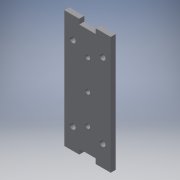
# Autodesk Inventor part: Tilt back support with counter balance option
Saved by Autodesk Inventor 2018 (Build 220112000, 112)
## iProperties
Created: 2018-06-26
Part Number: Tilt back support with counter balance option
Material: Generic
Document SubType Name: Modeling
Designer: Ajith Thomas
Density: 1 g/cm^3
Appearance: Default
Author: Ajith Thomas
Autodesk Inventor part; units mm, degrees
ref_plane "YZ Plane" through (0, 0, 0) normal (1, 0, 0) x (0, 1, 0)
ref_plane "XZ Plane" through (0, 0, 0) normal (0, 1, 0) x (-1, 0, 0)
ref_plane "XY Plane" through (0, 0, 0) normal (0, 0, 1) x (1, 0, 0)
sketch "Sketch1" plane through (0, 0, 0) normal (0, 0, 1) x (1, 0, 0)
  line L0 (5, 1.5) -> (-5, 1.5) projected
  line L1 (-5, 1.5) -> (-5, -1.5) projected
  line L2 (-5, -1.5) -> (5, -1.5) projected
  line L3 (5, -1.5) -> (5, 1.5) projected
  line L4 (5, -66.5) -> (-5, -66.5) projected
  line L5 (-5, -66.5) -> (-5, -69.5) projected
  line L6 (-5, -69.5) -> (5, -69.5) projected
  line L7 (5, -69.5) -> (5, -66.5) projected
  line L8 (14, -1.5) -> (14, 1.5) construction
  line L9 (-14, -1.5) -> (-14, 1.5) construction
  line L10 (-14, -69.5) -> (-14, -66.5) construction
  line L11 (14, -69.5) -> (14, -66.5) construction
  line L12 (14, 1.5) -> (-14, 1.5)
  line L13 (-14, 1.5) -> (-14, -69.5)
  line L14 (-14, -69.5) -> (14, -69.5)
  line L15 (14, -69.5) -> (14, 1.5)
  point P0 (0, 0)
  constraints: 8 end point, 2 parallel, 1 horizontal, 1 perpendicular
extrude "Extrusion1" add sketch "Sketch1" against normal blind 3 contours L12 L15 L14 L7 L4 L5 L13 L1 L2 L3
sketch "Sketch2" plane through (0, 0, 0) normal (0, 0, 1) x (1, 0, 0)
  line L0 (5, -66.5) -> (5, -69.5) construction
  line L1 (5, -69.5) -> (14, -69.5) construction
  line L2 (14, -69.5) -> (14, 1.5) construction
  line L3 (14, 1.5) -> (5, 1.5) construction
  line L4 (5, 1.5) -> (5, -1.5) construction
  line L5 (5, -1.5) -> (-5, -1.5) construction
  line L6 (-5, -1.5) -> (-5, 1.5) construction
  line L7 (-5, 1.5) -> (-14, 1.5) construction
  line L8 (-14, 1.5) -> (-14, -69.5) construction
  line L9 (-14, -69.5) -> (-5, -69.5) construction
  line L10 (-5, -69.5) -> (-5, -66.5) construction
  line L11 (-5, -66.5) -> (5, -66.5) construction
  line L12 (14, 1.5) -> (-14, -69.5) construction
  line L13 (5, -69.5) -> (14, -69.5) construction
  line L14 (-14, 1.5) -> (14, -69.5) construction
  circle A0 centre (0, -34) radius 1.5
  circle A1 centre (0, -16) radius 1.5
  circle A2 centre (0, -52) radius 1.5
  point P0 (0, 0)
  dimension "d2" = 3
  dimension "d3" = 3
  dimension "d4" = 3
  dimension "d5" = 18
  dimension "d6" = 18
  constraints: 4 end point, 3 centre point, 1 midpoint
  measures "d2" diameter of A0
  measures "d3" diameter of A1
  measures "d4" diameter of A2
  measures "d5" distance of A0.centre A1.centre
  measures "d6" distance of A2.centre A0.centre
extrude "Extrusion2" cut sketch "Sketch2" against normal blind 3
sketch "Sketch3" plane through (0, 0, -3) normal (0, 0, -1) x (-1, 0, 0)
  circle A0 centre (-9, -56.6) radius 1.8 projected
  circle A1 centre (-9, -11.4) radius 1.8 projected
  circle A2 centre (9, -11.4) radius 1.8 projected
  circle A3 centre (9, -56.6) radius 1.8 projected
  point P0 (0, 0)
extrude "Extrusion3" cut sketch "Sketch3" against normal blind 3
body "Solid1"
